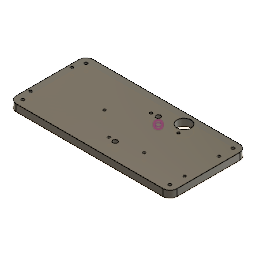
botenplata (Autodesk Fusion 360 design; units mm, degrees)
Autodesk Fusion 360 part; units mm, degrees
sketch "Sketch2" plane through (0, 0, 0) normal (0, 1, 0) x (1, 0, 0)
  line L0 (0, 0) -> (0, 110)
  line L1 (0, 0) -> (-230, 0)
  line L2 (-230, 0) -> (-230, 110)
  line L3 (-230, 110) -> (0, 110)
  dimension "d30" = 110
  dimension "d31" = 230
  dimension "d32" = 110
  measures "d31" distance of L0.start
  measures "d32" distance of L0.start
extrude "Extrude2" add sketch "Sketch2" along normal blind 10
sketch "Sketch3" plane through (0, 10, 0) normal (0, 1, 0) x (-1, 0, 0)
  line L0 (0, 0) -> (0, -110)
  line L1 (0, -110) -> (230, -110)
  line L2 (230, -110) -> (230, 0)
  line L3 (230, 0) -> (0, 0)
  circle A0 centre (102.5, -24.25) radius 3.25
  circle A1 centre (102.5, -85.75) radius 3.25
  dimension "d35" = 6.5
  dimension "d36" = 102.5
  dimension "d37" = 24.25
  dimension "d91" = 6.5
  dimension "d92" = 61.5
  measures "d35" diameter of A0
  measures "d37" distance of L3 L0.start
  measures "d91" diameter of A1
extrude "Extrude10" cut sketch "Sketch3" against normal blind 25 contours A1
extrude "Extrude3" cut sketch "Sketch3" against normal blind 50 contours A0
ref_plane "WorkPlane3" through (-115, 5, -55) normal (0, 0, 1) x (1, 0, 0)
fillet "Fillet1" radius 10 1 edges at (-230, 5, 0)
fillet "Fillet2" radius 10 3 edges at (-230, 5, -110) (0, 5, 0) (0, 5, -110)
sketch "Sketch4" plane through (0, 10, 0) normal (0, 1, 0) x (-1, 0, 0)
  arc A0 (0, -100) -> (10, -110) centre (10, -100) ccw
  line L0 (10, -110) -> (220, -110)
  arc A1 (220, -110) -> (230, -100) centre (220, -100) ccw
  line L1 (230, -100) -> (230, -10)
  arc A2 (230, -10) -> (220, 0) centre (220, -10) ccw
  line L2 (220, 0) -> (10, 0)
  arc A3 (10, 0) -> (0, -10) centre (10, -10) ccw
  line L3 (0, -10) -> (0, -100)
  circle A4 centre (102.5, -24.25) radius 3.25
  circle A5 centre (75, -95) radius 10
  circle A6 centre (102.5, -85.75) radius 3.25
  dimension "d44" = 20
  dimension "d90" = 3.5
  measures "d44" diameter of A5
extrude "Extrude4" cut sketch "Sketch4" against normal blind 45 contours A5
sketch "Sketch5" plane through (0, 10, 0) normal (0, 1, 0) x (-1, 0, 0)
  circle A0 centre (75, -95) radius 10
  arc A1 (0, -100) -> (10, -110) centre (10, -100) ccw
  line L0 (10, -110) -> (220, -110)
  arc A2 (220, -110) -> (230, -100) centre (220, -100) ccw
  line L1 (230, -100) -> (230, -10)
  arc A3 (230, -10) -> (220, 0) centre (220, -10) ccw
  line L2 (220, 0) -> (10, 0)
  arc A4 (10, 0) -> (0, -10) centre (10, -10) ccw
  line L3 (0, -10) -> (0, -100)
  circle A5 centre (102.5, -24.25) radius 3.25
  circle A6 centre (220, -100) radius 2
  circle A7 centre (102.5, -85.75) radius 3.25
  dimension "d47" = 4
  measures "d47" diameter of A6
extrude "Extrude5" cut sketch "Sketch5" against normal blind 23 contours A6
pattern_linear "R-Pattern1" count 2 spacing 90 along (0, 0, 1) of 1 faces at (-221.8794, 3.3333, -99.316)
pattern_linear "R-Pattern2" count 2 spacing 210 along (1, 0, 0) of 2 faces at (-221.8794, 3.3333, -99.316) (-219.0876, 6.6667, -11.7797)
sketch "Sketch7" plane through (0, 10, 0) normal (0, 1, 0) x (-1, 0, 0)
  circle A0 centre (10, -80) radius 1.75
  circle A1 centre (10, -31) radius 1.75
  circle A2 centre (68, -31) radius 1.75
  circle A3 centre (68, -80) radius 1.75
  dimension "d58" = 3.5
  dimension "d59" = 3.5
  dimension "d60" = 3.5
  dimension "d61" = 3.5
  dimension "d62" = 49
  dimension "d63" = 58
  dimension "d64" = 58
  dimension "d65" = 49
  measures "d58" diameter of A0
  measures "d59" diameter of A1
  measures "d60" diameter of A2
  measures "d61" diameter of A3
  measures "d63" distance of origin
  measures "d64" distance of origin
sketch "Sketch8" plane through (0, 10, 0) normal (0, 1, 0) x (-1, 0, 0)
  circle A0 centre (10, -10) radius 2
  circle A1 centre (10, -100) radius 2
  circle A2 centre (220, -10) radius 2
  circle A3 centre (220, -100) radius 2
  circle A4 centre (75, -95) radius 10
  arc A5 (0, -100) -> (10, -110) centre (10, -100) ccw
  line L0 (10, -110) -> (220, -110)
  arc A6 (220, -110) -> (230, -100) centre (220, -100) ccw
  line L1 (230, -100) -> (230, -10)
  arc A7 (230, -10) -> (220, 0) centre (220, -10) ccw
  line L2 (220, 0) -> (10, 0)
  arc A8 (10, 0) -> (0, -10) centre (10, -10) ccw
  line L3 (0, -10) -> (0, -100)
  circle A9 centre (102.5, -24.25) radius 3.25
  circle A10 centre (225, -85) radius 1.75
  circle A11 centre (225.0348, -26) radius 1.75
  circle A12 centre (112, -85) radius 1.75
  circle A13 centre (112.0348, -25) radius 1.75
  circle A14 centre (102.5, -85.75) radius 3.25
  dimension "d70" = 3.5
  dimension "d71" = 3.5
  dimension "d72" = 59
  dimension "d75" = 3.5
  dimension "d76" = 113
  dimension "d77" = 3.5
  dimension "d78" = 113
  measures "d70" diameter of A10
  measures "d71" diameter of A11
  measures "d75" diameter of A12
  measures "d77" diameter of A13
extrude "Extrude7" cut sketch "Sketch8" against normal blind 40 contours A10 | A11 | A12 | A13
extrude "Extrude8" cut sketch "Sketch7" against normal blind 30
sketch "Sketch9" plane through (0, 10, 0) normal (0, 1, 0) x (-1, 0, 0)
  circle A0 centre (10, -80) radius 1.75
  circle A1 centre (68, -31) radius 1.75
  circle A2 centre (68, -80) radius 1.75
  circle A3 centre (10, -31) radius 1.75
  circle A4 centre (225.0348, -26) radius 1.75
  circle A5 centre (112.0348, -25) radius 1.75
  circle A6 centre (225, -85) radius 1.75
  circle A7 centre (112, -85) radius 1.75
  circle A8 centre (10, -10) radius 2
  circle A9 centre (10, -100) radius 2
  circle A10 centre (220, -10) radius 2
  circle A11 centre (220, -100) radius 2
  circle A12 centre (75, -95) radius 10
  arc A13 (0, -100) -> (10, -110) centre (10, -100) ccw
  line L0 (10, -110) -> (220, -110)
  arc A14 (220, -110) -> (230, -100) centre (220, -100) ccw
  line L1 (230, -100) -> (230, -10)
  arc A15 (230, -10) -> (220, 0) centre (220, -10) ccw
  line L2 (220, 0) -> (10, 0)
  arc A16 (10, 0) -> (0, -10) centre (10, -10) ccw
  line L3 (0, -10) -> (0, -100)
  circle A17 centre (102.5, -24.25) radius 3.25
  circle A18 centre (102.5, -85.75) radius 3.25
sketch "Sketch10" plane through (0, 10, 0) normal (0, 1, 0) x (-1, 0, 0)
  circle A0 centre (149, -55.5) radius 1.75
  circle A1 centre (225.0348, -26) radius 1.75
  dimension "d83" = 3.5
  dimension "d84" = 76
  dimension "d85" = 29.5
  dimension "d86" = 30
  measures "d83" diameter of A0
extrude "Extrude9" cut sketch "Sketch10" against normal blind 55 contours A0
sketch "Sketch11" plane through (0, 10, 0) normal (0, 1, 0) x (-1, 0, 0)
  circle A0 centre (149, -55.5) radius 1.75
  circle A1 centre (10, -80) radius 1.75
  circle A2 centre (68, -31) radius 1.75
  circle A3 centre (68, -80) radius 1.75
  circle A4 centre (10, -31) radius 1.75
  circle A5 centre (225.0348, -26) radius 1.75
  circle A6 centre (112.0348, -25) radius 1.75
  circle A7 centre (225, -85) radius 1.75
  circle A8 centre (112, -85) radius 1.75
  circle A9 centre (10, -10) radius 2
  circle A10 centre (10, -100) radius 2
  circle A11 centre (220, -10) radius 2
  circle A12 centre (220, -100) radius 2
  circle A13 centre (75, -95) radius 10
  arc A14 (0, -100) -> (10, -110) centre (10, -100) ccw
  line L0 (10, -110) -> (220, -110)
  arc A15 (220, -110) -> (230, -100) centre (220, -100) ccw
  line L1 (230, -100) -> (230, -10)
  arc A16 (230, -10) -> (220, 0) centre (220, -10) ccw
  line L2 (220, 0) -> (10, 0)
  arc A17 (10, 0) -> (0, -10) centre (10, -10) ccw
  line L3 (0, -10) -> (0, -100)
  circle A18 centre (102.5, -24.25) radius 3.25
  circle A19 centre (102.5, -85.75) radius 3.25
sketch "Sketch12" plane through (0, 0, 0) normal (0, -1, 0) x (1, 0, 0)
  circle A0 centre (-149, -55.5) radius 1.75
  circle A1 centre (-10, -80) radius 1.75
  circle A2 centre (-68, -31) radius 1.75
  circle A3 centre (-68, -80) radius 1.75
  circle A4 centre (-10, -31) radius 1.75
  circle A5 centre (-225.0348, -26) radius 1.75
  circle A6 centre (-112.0348, -25) radius 1.75
  circle A7 centre (-225, -85) radius 1.75
  circle A8 centre (-112, -85) radius 1.75
  circle A9 centre (-10, -100) radius 2
  circle A10 centre (-10, -10) radius 2
  circle A11 centre (-220, -10) radius 2
  circle A12 centre (-220, -100) radius 2
  circle A13 centre (-75, -95) radius 10
  circle A14 centre (-102.5, -24.25) radius 3.25
  arc A15 (-10, -110) -> (0, -100) centre (-10, -100) ccw
  line L0 (0, -100) -> (0, -10)
  arc A16 (0, -10) -> (-10, 0) centre (-10, -10) ccw
  line L1 (-10, 0) -> (-220, 0)
  arc A17 (-220, 0) -> (-230, -10) centre (-220, -10) ccw
  line L2 (-230, -10) -> (-230, -100)
  arc A18 (-230, -100) -> (-220, -110) centre (-220, -100) ccw
  line L3 (-220, -110) -> (-10, -110)
  circle A19 centre (-102.5, -85.75) radius 3.25
extrude "Extrude6" [suppressed]
extrude "Extrude1" [suppressed]
ref_plane "WorkPlane1" through (-130, 5, -55) normal (0, 0, 1) x (1, 0, 0)
mirror "Mirror1" [suppressed]
ref_plane "WorkPlane2" through (-130, 5, -55) normal (1, 0, 0) x (0, 0, -1)
mirror "Mirror2" [suppressed]
